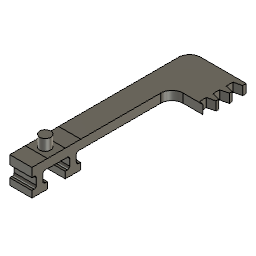
Left Claw (Autodesk Fusion 360 design; units mm, degrees)
Autodesk Fusion 360 part; units mm, degrees
sketch "Sketch1" plane through (0, 0, 0) normal (1, 0, 0) x (0, 1, 0)
  line L0 (0, 0) -> (0, 5) construction
  line L1 (0, 5) -> (3, 5) construction
  line L2 (3, 5) -> (3, 0) construction
  line L3 (3, 0) -> (0, 0) construction
  line L4 (0, 5) -> (-2, 5) construction
  line L5 (-2, 5) -> (-2, 9) construction
  line L6 (0, 0) -> (-2, 0) construction
  line L7 (-2, 0) -> (-2, -3) construction
  line L8 (-2, -3) -> (5, -3) construction
  line L9 (5, -3) -> (5, 0) construction
  line L10 (5, 0) -> (3, 0) construction
  line L11 (3, 5) -> (5, 5) construction
  line L12 (5, 5) -> (5, 9) construction
  line L13 (-2, 9) -> (5, 9) construction
  line L14 (-2, 5) -> (0, 5)
  line L15 (0, 5) -> (0, 0)
  line L16 (0, 0) -> (-2, 0)
  line L17 (-2, 0) -> (-2, -3)
  line L18 (-2, -3) -> (5, -3)
  line L19 (5, -3) -> (5, 0)
  line L20 (5, 0) -> (3, 0)
  line L21 (3, 0) -> (3, 5)
  line L22 (3, 5) -> (5, 5)
  line L23 (5, 5) -> (5, 9)
  line L24 (5, 9) -> (-2, 9)
  line L25 (-2, 9) -> (-2, 5)
  line L26 (-2, 5) -> (0, 5)
  line L27 (5, 9) -> (-2, 9)
  line L28 (-2, 0) -> (-2, -3)
  line L29 (3, 5) -> (5, 5) construction
  line L30 (5, 5) -> (5, 9) construction
  line L31 (5, 0) -> (3, 0)
  line L32 (-2, 0) -> (-2, -3) construction
  line L33 (5, 0) -> (3, 0) construction
  line L34 (-2, 9) -> (5, 9) construction
  line L35 (-2, -3) -> (5, -3) construction
  line L36 (-2, -3) -> (5, -3)
  line L37 (-2, 9) -> (-2, 5)
  line L38 (5, -3) -> (5, 0) construction
  line L39 (3, 5) -> (3, 0) construction
  line L40 (5, -3) -> (5, 0)
  line L41 (0, 0) -> (-2, 0)
  line L42 (3, 0) -> (3, 5)
  line L43 (0, 0) -> (-2, 0) construction
  line L44 (-2, 5) -> (-2, 9) construction
  line L45 (0, 5) -> (3, 5) construction
  line L46 (3, 5) -> (5, 5)
  line L47 (5, 5) -> (5, 9)
  line L48 (0, 0) -> (0, 5) construction
  line L49 (3, 0) -> (0, 0) construction
  line L50 (0, 5) -> (-2, 5) construction
  line L51 (0, 5) -> (0, 0)
  line L52 (13, 5) -> (15, 5)
  line L53 (20, 9) -> (13, 9)
  line L54 (13, 0) -> (13, -3)
  line L55 (18, 5) -> (20, 5) construction
  line L56 (20, 5) -> (20, 9) construction
  line L57 (20, 0) -> (18, 0)
  line L58 (13, 0) -> (13, -3) construction
  line L59 (20, 0) -> (18, 0) construction
  line L60 (13, 9) -> (20, 9) construction
  line L61 (13, -3) -> (20, -3) construction
  line L62 (13, -3) -> (20, -3)
  line L63 (13, 9) -> (13, 5)
  line L64 (20, -3) -> (20, 0) construction
  line L65 (18, 5) -> (18, 0) construction
  line L66 (20, -3) -> (20, 0)
  line L67 (15, 0) -> (13, 0)
  line L68 (18, 0) -> (18, 5)
  line L69 (15, 0) -> (13, 0) construction
  line L70 (13, 5) -> (13, 9) construction
  line L71 (15, 5) -> (18, 5) construction
  line L72 (18, 5) -> (20, 5)
  line L73 (20, 5) -> (20, 9)
  line L74 (15, 0) -> (15, 5) construction
  line L75 (18, 0) -> (15, 0) construction
  line L76 (15, 5) -> (13, 5) construction
  line L77 (15, 5) -> (15, 0)
  point P0 (15, 0)
  dimension "d1" = 5
  dimension "d2" = 3
  dimension "d3" = 2
  dimension "d4" = 4
  dimension "d5" = 3
  dimension "d6" = 2
  dimension "d7" = 4
  dimension "d8" = 5
  dimension "d9" = 3
  dimension "d10" = 2
  dimension "d11" = 4
  dimension "d12" = 3
  dimension "d13" = 2
  dimension "d14" = 4
  dimension "d15" = 5
  dimension "d16" = 3
  dimension "d17" = 2
  dimension "d18" = 4
  dimension "d19" = 3
  dimension "d20" = 2
  dimension "d21" = 4
  constraint coincident L0.start L3.end
  constraint vertical L0
  constraint perpendicular L0 L1
  constraint perpendicular L1 L2
  constraint perpendicular L0 L3
  constraint perpendicular L0 L4
  constraint perpendicular L4 L5
  constraint perpendicular L5 L6
  constraint perpendicular L6 L7
  constraint perpendicular L7 L8
  constraint perpendicular L8 L9
  constraint perpendicular L2 L10
  constraint perpendicular L2 L11
  constraint perpendicular L11 L12
  constraint vertical L48
  constraint perpendicular L45 L48
  constraint perpendicular L39 L45
  constraint perpendicular L48 L49
  constraint perpendicular L48 L50
  constraint perpendicular L44 L50
  constraint perpendicular L43 L44
  constraint perpendicular L32 L43
  constraint perpendicular L32 L35
  constraint perpendicular L35 L38
  constraint perpendicular L33 L39
  constraint perpendicular L29 L39
  constraint perpendicular L29 L30
  constraint coincident P0 L67.start
  constraint vertical L74
  constraint perpendicular L71 L74
  constraint perpendicular L65 L71
  constraint perpendicular L74 L75
  constraint perpendicular L74 L76
  constraint perpendicular L70 L76
  constraint perpendicular L69 L70
  constraint perpendicular L58 L69
  constraint perpendicular L58 L61
  constraint perpendicular L61 L64
  constraint perpendicular L59 L65
  constraint perpendicular L55 L65
  constraint perpendicular L55 L56
  measures "d1" distance of L0.start L0.end
  measures "d2" distance of L0.end L1.end
  measures "d3" distance of L0.end L4.end
  measures "d4" distance of L4.end L5.end
  measures "d5" distance of L6.end L7.end
  measures "d6" distance of L1.end L11.end
  measures "d7" distance of L11.end L12.end
  measures "d8" distance of L0.end L0.start
  measures "d9" distance of L0.end L1.end
  measures "d10" distance of L0.end L4.end
  measures "d11" distance of L4.end L5.end
  measures "d12" distance of L7.end L6.end
  measures "d13" distance of L11.end L1.end
  measures "d14" distance of L11.end L12.end
  measures "d15" distance of L52.end P0
  measures "d16" distance of L52.end L55.start
  measures "d17" distance of L52.end L52.start
  measures "d18" distance of L52.start L53.end
  measures "d19" distance of L54.end L54.start
  measures "d20" distance of L55.end L55.start
  measures "d21" distance of L55.end L53.start
extrude "Extrude1" add sketch "Sketch1" along normal blind 10 makes body 1 at (6.6667, 0.3333, -3) makes body 2 at (3.3333, 15.3333, -3)
extrude "Extrude2" add 1 faces at (3.3333, 5, 6.3333) along direction (0, 1, 0) blind 8 on bodies 1 bodies 1 2
fillet "Fillet1" radius 1 1 edges at (5, 18, 5) on bodies 1
fillet "Fillet2" radius 1 1 edges at (5, 18, 0) on bodies 1
fillet "Fillet3" radius 1 1 edges at (5, 15, 0) on bodies 1
fillet "Fillet4" radius 1 1 edges at (5, 15, 5) on bodies 1
fillet "Fillet5" radius 1 1 edges at (5, 3, 0) on bodies 1
fillet "Fillet6" radius 1 1 edges at (5, 0, 0) on bodies 1
fillet "Fillet7" radius 1 1 edges at (5, 0, 5) on bodies 1
fillet "Fillet8" radius 1 1 edges at (5, 3, 5) on bodies 1
extrude "Extrude3" add 1 faces at (3.3333, 20, 6.3333) along direction (0, 1, 0) blind 59 on bodies 1 bodies 1
sketch "Sketch2" plane through (0, 0, 9) normal (0, 0, 1) x (-1, 0, 0)
  line L0 (0, -5) -> (-10, -5)
  line L1 (-10, -5) -> (-10, -13)
  line L2 (-10, -13) -> (0, -13)
  line L3 (0, -13) -> (0, -5)
  line L4 (-5, -13) -> (-5, -9) construction
  circle A0 centre (-5, -9) radius 2.5
  dimension "d44" = 5
  constraint midpoint L2 L4.start
  constraint perpendicular L0 L4
  constraint coincident L4.end A0.centre
  measures "d44" diameter of A0
extrude "Extrude4" add sketch "Sketch2" along normal blind 5 contours A0 bodies 1
sketch "Sketch3" plane through (10, 0, 0) normal (1, 0, 0) x (0, 1, 0)
  line L0 (0, 4) -> (0, 1)
  arc A0 (-1, 0) -> (0, 1) centre (-1, 1) ccw
  line L1 (-1, 0) -> (-2, 0)
  line L2 (-2, 0) -> (-2, -3)
  line L3 (-2, -3) -> (5, -3)
  line L4 (5, -3) -> (5, 0)
  line L5 (5, 0) -> (4, 0)
  arc A1 (3, 1) -> (4, 0) centre (4, 1) ccw
  line L6 (3, 1) -> (3, 4)
  arc A2 (4, 5) -> (3, 4) centre (4, 4) ccw
  line L7 (4, 5) -> (14, 5)
  arc A3 (15, 4) -> (14, 5) centre (14, 4) ccw
  line L8 (15, 4) -> (15, 1)
  arc A4 (14, 0) -> (15, 1) centre (14, 1) ccw
  line L9 (14, 0) -> (13, 0)
  line L10 (13, 0) -> (13, -3)
  line L11 (13, -3) -> (20, -3)
  line L12 (20, -3) -> (20, 0)
  line L13 (20, 0) -> (19, 0)
  arc A5 (18, 1) -> (19, 0) centre (19, 1) ccw
  line L14 (18, 1) -> (18, 4)
  arc A6 (19, 5) -> (18, 4) centre (19, 4) ccw
  line L15 (19, 5) -> (79, 5)
  line L16 (79, 5) -> (79, 9)
  line L17 (79, 9) -> (20, 9)
  line L18 (20, 9) -> (13, 9)
  line L19 (13, 9) -> (5, 9)
  line L20 (5, 9) -> (-2, 9)
  line L21 (-2, 9) -> (-2, 5)
  line L22 (-2, 5) -> (-1, 5)
  arc A7 (0, 4) -> (-1, 5) centre (-1, 4) ccw
  line L23 (79, 5) -> (61, 5)
  line L24 (61, 5) -> (61, 9)
  line L25 (61, 9) -> (79, 9)
  line L26 (79, 9) -> (79, 5)
  dimension "d47" = 18
  constraint horizontal L23
  constraint vertical L24
  constraint horizontal L25
  constraint vertical L26
  constraint coincident L15.end L16.start
  measures "d47" distance of L15.end L23.end
extrude "Extrude5" add sketch "Sketch3" along normal blind 14 contours L15 L16 L17 L23 L24 L25 L26 bodies 1
fillet "Fillet9" radius 5 1 edges at (10, 61, 7) on bodies 1
fillet "Fillet10" radius 5 1 edges at (0, 79, 7) on bodies 1
sketch "Sketch4" plane through (0, 0, 9) normal (0, 0, 1) x (-1, 0, 0)
  arc A0 (-5, -79) -> (0, -74) centre (-5, -74) ccw
  line L0 (0, -74) -> (0, -20)
  line L1 (0, -20) -> (-10, -20)
  line L2 (-10, -20) -> (-10, -56)
  arc A1 (-15, -61) -> (-10, -56) centre (-15, -56) ccw
  line L3 (-15, -61) -> (-24, -61)
  line L4 (-24, -61) -> (-24, -79)
  line L5 (-24, -79) -> (-5, -79)
  line L6 (-22, -79) -> (-26, -79) construction
  line L7 (-26, -79) -> (-26, -61) construction
  line L8 (-26, -61) -> (-22, -61) construction
  line L9 (-22, -61) -> (-22, -79) construction
  line L10 (-26, -79) -> (-26, -77) construction
  line L11 (-26, -77) -> (-22, -76) construction
  line L12 (-22, -74) -> (-26, -73) construction
  line L13 (-26, -71) -> (-22, -70) construction
  line L14 (-22, -68) -> (-26, -67) construction
  line L15 (-26, -65) -> (-22, -64) construction
  line L16 (-22, -62) -> (-26, -61) construction
  line L17 (-26, -77) -> (-26, -77.5) construction
  line L18 (-22, -76) -> (-22, -76.5) construction
  line L19 (-26, -79) -> (-25.5, -79) construction
  line L20 (-26, -77.5) -> (-22, -76.5) construction
  line L21 (-25.5, -79) -> (-25.5, -77.375) construction
  line L22 (-26, -73) -> (-26, -72.5) construction
  line L23 (-22, -73.5) -> (-26, -72.5) construction
  line L24 (-26, -71.5) -> (-22, -70.5) construction
  line L25 (-22, -67.5) -> (-26, -66.5) construction
  line L26 (-22, -64.5) -> (-26, -65.5) construction
  line L27 (-22, -61.5) -> (-26, -60.5) construction
  line L28 (-25.5009, -60.6248) -> (-25.5009, -61.1248) construction
  line L29 (-25.5, -79) -> (-25.5, -77.375)
  line L30 (-25.5, -77.375) -> (-22, -76.5)
  line L31 (-25.5, -72.625) -> (-25.5, -71.375)
  line L32 (-22, -73.5) -> (-25.5, -72.625)
  line L33 (-25.5, -71.375) -> (-22, -70.5)
  line L34 (-25.5022, -66.6245) -> (-25.5022, -65.3756)
  line L35 (-22, -67.5) -> (-25.5022, -66.6245)
  line L36 (-22, -64.5) -> (-25.5022, -65.3756)
  line L37 (-22, -61.5) -> (-24.0719, -61)
  line L38 (-25.5, -79) -> (-22, -79)
  line L39 (-22, -79) -> (-22, -76.5)
  line L40 (-22, -73.5) -> (-22, -70.5)
  line L41 (-22, -67.5) -> (-22, -64.5)
  line L42 (-22, -61.5) -> (-22, -61)
  line L43 (-22, -61) -> (-24, -61)
  line L44 (-22, -70.5) -> (-22, -67.5)
  line L45 (-24, -71) -> (-24, -67)
  line L46 (-24, -65) -> (-24, -61)
  line L47 (-22, -64.5) -> (-22, -61.5)
  line L48 (-22, -76.5) -> (-22, -73.5)
  line L49 (-24, -77) -> (-24, -73)
  dimension "d54" = 0.5
  dimension "d55" = 0.5
  constraint horizontal L6
  constraint vertical L7
  constraint horizontal L8
  constraint vertical L9
  constraint coincident L5 L6.start
  constraint coincident L7 L10.end
  constraint coincident L9 L11.end
  constraint coincident L9 L12.start
  constraint coincident L7 L12.end
  constraint coincident L7 L13.start
  constraint midpoint L9 L13.end
  constraint parallel L11 L13
  constraint coincident L9 L14.start
  constraint coincident L7 L14.end
  constraint parallel L12 L14
  constraint coincident L7 L15.start
  constraint coincident L9 L15.end
  constraint parallel L13 L15
  constraint coincident L9 L16.start
  constraint parallel L14 L16
  constraint parallel L7 L17
  constraint parallel L9 L18
  constraint coincident L6 L19.end
  constraint coincident L20 L21.end
  constraint perpendicular L6 L21
  constraint coincident L7 L22.end
  constraint coincident L9 L23.start
  constraint coincident L7 L24.start
  constraint coincident L9 L24.end
  constraint coincident L9 L25.start
  constraint coincident L7 L25.end
  constraint parallel L23 L25
  constraint coincident L9 L26.start
  constraint coincident L7 L26.end
  constraint parallel L24 L26
  constraint coincident L9 L27.start
  constraint parallel L16 L27
  constraint coincident L27 L28.start
  constraint coincident L16 L28.end
  constraint perpendicular L8 L28
  constraint coincident L23 L31.start
  constraint coincident L24 L31.end
  constraint parallel L9 L31
  constraint parallel L24 L33
  constraint coincident L25 L34.start
  constraint coincident L26 L34.end
  constraint vertical L34
  constraint coincident L8 L37.end
  constraint parallel L9 L40
  constraint coincident L3.end L4.start
  constraint midpoint L24 L45.start
  constraint midpoint L25 L45.end
  constraint midpoint L26 L46.start
  constraint midpoint L20 L49.start
  constraint midpoint L23 L49.end
  measures "d54" distance of L10.end L17.end
  measures "d55" distance of L11.end L18.end
extrude "Extrude6" add sketch "Sketch4" against normal blind 4 contours L4 L29 L30 L38 | L4 L31 L32 L33 | L4 L34 L35 L36 bodies 1
extrude "Extrude7" cut sketch "Sketch4" against normal blind 4 contours L4 L30 L32 L48 L49 | L4 L33 L35 L44 L45 | L4 L36 L37 L46 L47 bodies 1
